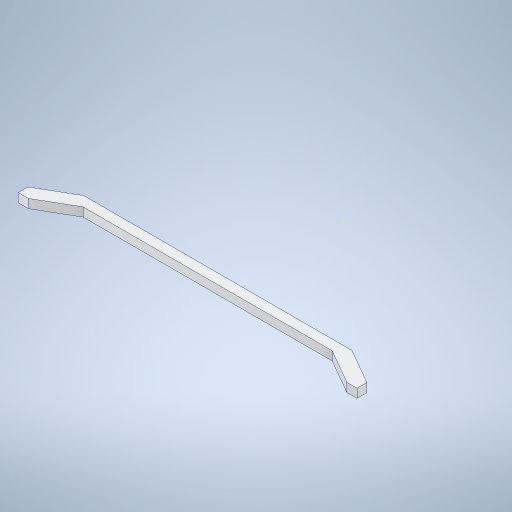
# Autodesk Inventor part: UcreplenieX
Saved by Autodesk Inventor 2024 (Build 280153000, 153)
## iProperties
Created: 2023-11-16
Part Number: UcreplenieX
Material: Aluminum 6061
Document SubType Name: Modeling
Designer: KirikDK
Mass: 2320.2 g
Surface Area: 1240.47 cm^2
Volume: 859.335 cm^3
Density: 2.7 g/cm^3
Appearance: Aluminum - Flat
Author: KirikDK
Autodesk Inventor part; units mm, degrees
ref_plane "YZ Plane" through (0, 0, 0) normal (1, 0, 0) x (0, 1, 0)
ref_plane "XZ Plane" through (0, 0, 0) normal (0, 1, 0) x (-1, 0, 0)
ref_plane "XY Plane" through (0, 0, 0) normal (0, 0, 1) x (1, 0, 0)
sketch "Sketch1" plane through (0, 0, 0) normal (0, 1, 0) x (-1, 0, 0)
  line L0 (555.2926, 403.499) -> (-444.7074, 403.499)
  line L1 (-444.7074, 403.499) -> (-444.7074, 314.499)
  line L2 (-444.7074, 314.499) -> (555.2926, 314.499)
  line L3 (555.2926, 314.499) -> (555.2926, 403.499)
  line L4 (423.1016, 344.499) -> (-312.5164, 344.499)
  line L5 (-444.7074, 403.499) -> (-414.7074, 403.499)
  line L6 (-414.7074, 403.499) -> (-414.7074, 374.7123)
  line L7 (-414.7074, 374.7123) -> (-444.7074, 374.7123)
  line L8 (-444.7074, 374.7123) -> (-444.7074, 403.499)
  line L9 (555.2926, 403.499) -> (525.2926, 403.499)
  line L10 (525.2926, 403.499) -> (525.2926, 374.7123)
  line L11 (525.2926, 374.7123) -> (555.2926, 374.7123)
  line L12 (555.2926, 374.7123) -> (555.2926, 403.499)
  line L13 (525.2926, 403.499) -> (423.1016, 344.499)
  line L14 (-414.7074, 403.499) -> (-312.5164, 344.499)
  line L15 (-444.7074, 374.7123) -> (-340.4148, 314.499)
  line L16 (555.2926, 374.7123) -> (451, 314.499)
  point P0 (0, 0)
  point P1 (555.2926, 368.7138)
  point P2 (522.9975, 314.499)
  point P3 (-444.7074, 354.0015)
  point P4 (-397.9975, 314.499)
  point P5 (525.2926, 403.499)
  point P6 (525.2926, 403.499)
  dimension "d0" = 1000
  dimension "d5" = 30
  dimension "d11" = 89
  dimension "d12" = 30
  dimension "d13" = 30
  dimension "d17" = 60
  dimension "d18" = 60
  constraints: 34 end point, 8 parallel, 7 point on line, 4 horizontal, 3 perpendicular
  measures "d0" distance of L1.end L2.end
  measures "d5" distance between parallel lines of L2 L4
  measures "d11" distance of L2.end L0.start
  measures "d12" distance of L6.end L7.end
  measures "d13" distance of L10.end L11.end
  measures "d17" angle of L6 L14
  measures "d18" angle of L10 L13
extrude "Extrusion1" add sketch "Sketch1" along normal blind 26 contours L3 L11 L10 L0 | L10 L11 L16 L2 L15 L7 L6 L14 L4 L13 | L6 L7 L1 L0
sketch "Sketch2" plane through (0, 26, 0) normal (0, 1, 0) x (1, 0, 0)
  point P0 (0, 0)
body "Solid1"
